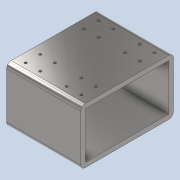
# Autodesk Inventor part: 3in x 5in Steel Rectangular Tubing 4in long
Saved by Autodesk Inventor 2022 (Build 260153000, 153)
## iProperties
Created: 2021-10-11
Part Number: 3in x 5in Steel Rectangular Tubing 4in long
Material: Generic
Document SubType Name: Modeling
Designer: Coy
Density: 1 g/cm^3
Appearance: Galvanized
Author: Coy
Autodesk Inventor part; units mm, degrees
ref_plane "YZ Plane" through (0, 0, 0) normal (1, 0, 0) x (0, 1, 0)
ref_plane "XZ Plane" through (0, 0, 0) normal (0, 1, 0) x (-1, 0, 0)
ref_plane "XY Plane" through (0, 0, 0) normal (0, 0, 1) x (1, 0, 0)
sketch "Sketch1" plane through (0, 0, 0) normal (1, 0, 0) x (0, 1, 0)
  line L0 (6.35, 0) -> (69.85, 0)
  line L1 (76.2, -6.35) -> (76.2, -120.65)
  line L2 (69.85, -127) -> (6.35, -127)
  line L3 (0, -120.65) -> (0, -6.35)
  arc A0 (76.2, -6.35) -> (69.85, 0) centre (69.85, -6.35) ccw
  arc A1 (69.85, -127) -> (76.2, -120.65) centre (69.85, -120.65) ccw
  arc A2 (0, -120.65) -> (6.35, -127) centre (6.35, -120.65) ccw
  arc A3 (6.35, 0) -> (0, -6.35) centre (6.35, -6.35) ccw
  line L4 (69.85, -120.65) -> (69.85, -6.35)
  line L5 (69.85, -6.35) -> (6.35, -6.35)
  line L6 (6.35, -6.35) -> (6.35, -120.65)
  line L7 (6.35, -120.65) -> (69.85, -120.65)
  point P0 (0, 0)
  point P1 (76.2, -127)
  point P2 (76.2, 0)
  point P3 (0, -127)
  dimension "d0" = 76.2
  dimension "d1" = 127
  dimension "d2" = 6.35
  dimension "d3" = 6.35
  dimension "d4" = 6.35
  constraints: 16 end point, 8 point on circle, 8 point on line, 8 tangent, 4 centre point, 4 parallel, 2 equal radius, 2 perpendicular, 1 horizontal, 3 other
  measures "d0" distance of point (76.2, -127) point (0, -127)
  measures "d1" distance of point (76.2, 0) point (76.2, -127)
  measures "d2" radius of A0
  measures "d3" radius of A3
  measures "d4" distance between parallel lines of L1 L4
extrude "Extrusion1" add sketch "Sketch1" against normal blind 101.6
sketch "Sketch2" plane through (0, 76.2, -6.35) normal (0, 1, 0) x (1, 0, 0)
  line L0 (0, 0) -> (0, 114.3) construction
  line L1 (0, 57.15) -> (-101.6, 57.15) construction
  line L2 (-101.6, 114.3) -> (-101.6, 0) construction
  line L3 (0, 83.65) -> (-45.4, 83.65) construction
  line L4 (-45.4, 83.65) -> (-45.4, 110.65) construction
  line L5 (-45.4, 110.65) -> (0, 110.65) construction
  line L6 (0, 110.65) -> (0, 83.65) construction
  line L7 (-32.7, 107.15) -> (-12.7, 107.15) construction
  line L8 (-12.7, 107.15) -> (-12.7, 87.15) construction
  line L9 (-12.7, 87.15) -> (-32.7, 87.15) construction
  line L10 (-32.7, 87.15) -> (-32.7, 107.15) construction
  line L11 (-32.7, 107.15) -> (-32.7, 110.65) construction
  line L12 (-32.7, 107.15) -> (-45.4, 107.15) construction
  line L13 (-12.7, 87.15) -> (-12.7, 83.65) construction
  line L14 (-12.7, 87.15) -> (0, 87.15) construction
  circle A0 centre (-32.7, 107.15) radius 1.6
  circle A1 centre (-12.7, 107.15) radius 1.6
  circle A2 centre (-12.7, 87.15) radius 1.6
  circle A3 centre (-32.7, 87.15) radius 1.6
  line L15 (0, 114.3) -> (0, 0) construction
  line L16 (-50.8, 57.15) -> (-50.8, 128.3257) construction
  line L17 (-101.6, 83.65) -> (-56.2, 83.65) construction
  line L18 (-56.2, 83.65) -> (-56.2, 110.65) construction
  line L19 (-56.2, 110.65) -> (-101.6, 110.65) construction
  line L20 (-101.6, 110.65) -> (-101.6, 83.65) construction
  line L21 (-68.9, 107.15) -> (-88.9, 107.15) construction
  line L22 (-88.9, 107.15) -> (-88.9, 87.15) construction
  line L23 (-88.9, 87.15) -> (-68.9, 87.15) construction
  line L24 (-68.9, 87.15) -> (-68.9, 107.15) construction
  line L25 (-68.9, 107.15) -> (-68.9, 110.65) construction
  line L26 (-68.9, 107.15) -> (-56.2, 107.15) construction
  line L27 (-88.9, 87.15) -> (-88.9, 83.65) construction
  line L28 (-88.9, 87.15) -> (-101.6, 87.15) construction
  circle A4 centre (-68.9, 107.15) radius 1.6
  circle A5 centre (-88.9, 107.15) radius 1.6
  circle A6 centre (-88.9, 87.15) radius 1.6
  circle A7 centre (-68.9, 87.15) radius 1.6
  line L29 (0, 30.65) -> (-45.4, 30.65) construction
  line L30 (-45.4, 30.65) -> (-45.4, 3.65) construction
  line L31 (-45.4, 3.65) -> (0, 3.65) construction
  line L32 (0, 3.65) -> (0, 30.65) construction
  line L33 (-32.7, 7.15) -> (-12.7, 7.15) construction
  line L34 (-12.7, 7.15) -> (-12.7, 27.15) construction
  line L35 (-12.7, 27.15) -> (-32.7, 27.15) construction
  line L36 (-32.7, 27.15) -> (-32.7, 7.15) construction
  line L37 (-32.7, 7.15) -> (-32.7, 3.65) construction
  line L38 (-32.7, 7.15) -> (-45.4, 7.15) construction
  line L39 (-12.7, 27.15) -> (-12.7, 30.65) construction
  line L40 (-12.7, 27.15) -> (0, 27.15) construction
  circle A8 centre (-32.7, 7.15) radius 1.6
  circle A9 centre (-12.7, 7.15) radius 1.6
  circle A10 centre (-12.7, 27.15) radius 1.6
  circle A11 centre (-32.7, 27.15) radius 1.6
  line L41 (-68.9, 7.15) -> (-88.9, 7.15) construction
  line L42 (-88.9, 27.15) -> (-68.9, 27.15) construction
  line L43 (-88.9, 27.15) -> (-88.9, 30.65) construction
  line L44 (-88.9, 7.15) -> (-88.9, 27.15) construction
  circle A12 centre (-88.9, 27.15) radius 1.6
  circle A13 centre (-88.9, 7.15) radius 1.6
  line L45 (-101.6, 30.65) -> (-56.2, 30.65) construction
  line L46 (-101.6, 3.65) -> (-101.6, 30.65) construction
  line L47 (-88.9, 27.15) -> (-101.6, 27.15) construction
  line L48 (-56.2, 3.65) -> (-101.6, 3.65) construction
  line L49 (-68.9, 27.15) -> (-68.9, 7.15) construction
  line L50 (-68.9, 7.15) -> (-68.9, 3.65) construction
  circle A14 centre (-68.9, 7.15) radius 1.6
  circle A15 centre (-68.9, 27.15) radius 1.6
  line L51 (-56.2, 30.65) -> (-56.2, 3.65) construction
  line L52 (-68.9, 7.15) -> (-56.2, 7.15) construction
  point P0 (0, -6.35)
  dimension "d7" = 45.4
  dimension "d8" = 27
  dimension "d9" = 20
  dimension "d10" = 20
  dimension "d11" = 3.2
  dimension "d12" = 3.2
  dimension "d13" = 3.2
  dimension "d14" = 3.2
  dimension "d15" = 100
  constraints: 100 end point, 48 symmetric about line, 17 point on line, 16 centre point, 16 coincident, 6 parallel, 6 perpendicular, 3 midpoint, 2 horizontal, 1 vertical, 12 other
  measures "d7" distance of L4.end L5.end
  measures "d8" distance of L3.end L4.end
  measures "d9" distance of L8.end L9.end
  measures "d10" distance of L7.end L8.end
  measures "d11" diameter of A0
  measures "d12" diameter of A1
  measures "d13" diameter of A3
  measures "d14" diameter of A2
  measures "d15" diameter of L7 L1
extrude "Extrusion2" cut sketch "Sketch2" against normal up to next
equation "\"d12\" = d11"
equation "\"d13\" = d11"
equation "\"d14\" = d11"
equation "\"d16\" = d12"
body "Solid1"
